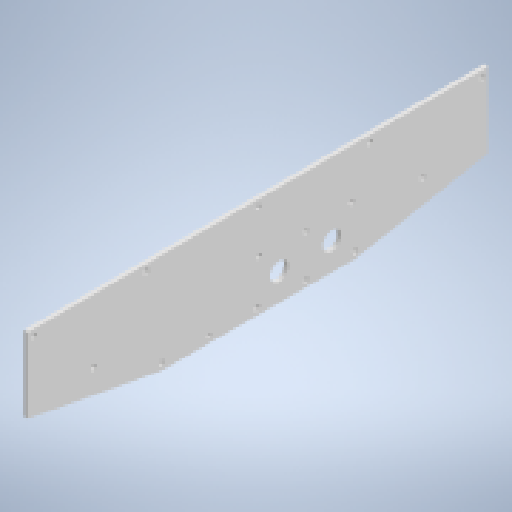
# Autodesk Inventor part: InsideChassiPlate3.0
Saved by Autodesk Inventor 2023 (Build 270158000, 158)
## iProperties
Created: 2022-09-18
Part Number: InsideChassiPlate3.0
Material: Generic
Document SubType Name: Modeling
Designer: deli
Density: 1 g/cm^3
Appearance: Default
Author: deli
Autodesk Inventor part; units mm, degrees
ref_plane "YZ Plane" through (0, 0, 0) normal (1, 0, 0) x (0, 1, 0)
ref_plane "XZ Plane" through (0, 0, 0) normal (0, 1, 0) x (-1, 0, 0)
ref_plane "XY Plane" through (0, 0, 0) normal (0, 0, 1) x (1, 0, 0)
sketch "Sketch1" plane through (0, 0, 0) normal (1, 0, 0) x (0, 1, 0)
  circle A0 centre (168.017, -47.9087) radius 7 construction
  circle A1 centre (168.017, -88.0464) radius 7 construction
  line L0 (147.267, 41.7418) -> (147.267, -105.149) projected
  arc A2 (147.267, -105.149) -> (147.3544, -106.0799) centre (152.267, -105.149) ccw projected
  line L1 (147.3544, -106.0799) -> (166.4208, -206.7036) projected
  line L2 (166.4208, -206.7036) -> (253.267, -206.7036) projected
  line L3 (253.267, -206.7036) -> (253.267, 143.2964) projected
  line L4 (253.267, 143.2964) -> (166.4208, 143.2964) projected
  line L5 (166.4208, 143.2964) -> (147.3544, 42.6727) projected
  arc A3 (147.3544, 42.6727) -> (147.267, 41.7418) centre (152.267, 41.7418) ccw projected
  circle A4 centre (152.267, 5.4679) radius 2 projected
  circle A5 centre (218.267, 53.2964) radius 2 projected
  circle A6 centre (243.267, -56.7036) radius 1.6 projected
  circle A7 centre (218.267, -116.7036) radius 2 projected
  circle A8 centre (218.267, -201.7036) radius 2 projected
  circle A9 centre (186.186, -102.5532) radius 2 projected
  circle A10 centre (152.267, -30.806) radius 2 projected
  circle A11 centre (151.883, -67.9775) radius 2 projected
  circle A12 centre (184.1509, -67.9775) radius 2 projected
  circle A13 centre (168.017, -88.0464) radius 7 projected
  circle A14 centre (168.017, -47.9087) radius 7 projected
  circle A15 centre (175.267, -156.7036) radius 2 projected
  circle A16 centre (175.267, 93.2964) radius 2 projected
  circle A17 centre (218.267, 138.2964) radius 2 projected
  circle A18 centre (185.4689, -32.5466) radius 2 projected
  circle A19 centre (243.267, 128.2964) radius 1.6 projected
  circle A20 centre (218.267, -31.7036) radius 2 projected
  circle A21 centre (152.267, 41.7418) radius 2 projected
  circle A22 centre (152.267, -105.149) radius 2 projected
  line L6 (223.267, 143.2964) -> (223.267, -206.7036)
  point P0 (0, 0)
  point P1 (168.017, -138.0464)
  point P2 (168.017, -97.9204)
  dimension "d5" = 30
  constraints: 2 end point, 2 point on line, 1 perpendicular
  measures "d5" distance between parallel lines of L3 L6
extrude "Extrusion1" add sketch "Sketch1" along normal blind 3.175 contours A3 L5 L4 L6 L2 L1 A2 L0
body "Solid1"
